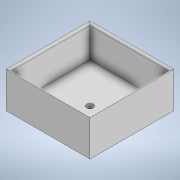
# Autodesk Inventor part: KwadratP
Saved by Autodesk Inventor 2020.3 (Build 243373000, 373)
## iProperties
Created: 2021-05-21
Part Number: KwadratP
Material: Generic
Document SubType Name: Modeling
Designer: patry
Density: 1 g/cm^3
Appearance: Default
Author: patry
Autodesk Inventor part; units mm, degrees
ref_plane "YZ Plane" through (0, 0, 0) normal (1, 0, 0) x (0, 1, 0)
ref_plane "XZ Plane" through (0, 0, 0) normal (0, 1, 0) x (-1, 0, 0)
ref_plane "XY Plane" through (0, 0, 0) normal (0, 0, 1) x (1, 0, 0)
sketch "Sketch1" plane through (0, 0, 0) normal (0, 1, 0) x (-1, 0, 0)
  line L0 (-52.5, -52.5) -> (52.5, -52.5)
  line L1 (52.5, -52.5) -> (52.5, 52.5)
  line L2 (52.5, 52.5) -> (-52.5, 52.5)
  line L3 (-52.5, 52.5) -> (-52.5, -52.5)
  line L4 (-52.5, -52.5) -> (52.5, 52.5) construction
  line L5 (52.5, -52.5) -> (-52.5, 52.5) construction
  point P0 (0, 0)
  constraints: 12 end point, 2 parallel, 1 horizontal, 1 perpendicular
extrude "Extrusion1" add sketch "Sketch1" along normal blind 5
sketch "Sketch4" plane through (0, 5, 0) normal (0, 1, 0) x (1, 0, 0)
  line L0 (-52.5, 52.5) -> (-52.5, -52.5) projected
  line L1 (52.5, 52.5) -> (-52.5, 52.5)
  line L2 (-52.5, 52.5) -> (-52.5, -52.5)
  line L3 (-52.5, -52.5) -> (52.5, -52.5)
  line L4 (52.5, -52.5) -> (52.5, 52.5)
  line L5 (52.5, 52.5) -> (-52.5, -52.5) construction
  line L6 (-52.5, 52.5) -> (52.5, -52.5) construction
  line L7 (50, 50) -> (-50, 50)
  line L8 (-50, 50) -> (-50, -50)
  line L9 (-50, -50) -> (50, -50)
  line L10 (50, -50) -> (50, 50)
  line L11 (50, 50) -> (-50, -50) construction
  line L12 (-50, 50) -> (50, -50) construction
  line L13 (52.5, 52.5) -> (-52.5, 52.5)
  line L14 (-52.5, 52.5) -> (-52.5, -52.5)
  line L15 (-52.5, -52.5) -> (52.5, -52.5)
  line L16 (52.5, -52.5) -> (52.5, 52.5)
  line L17 (52.5, 52.5) -> (-52.5, -52.5) construction
  line L18 (-52.5, 52.5) -> (52.5, -52.5) construction
  point P0 (0, 0)
  constraints: 36 end point, 6 midpoint, 6 parallel, 3 horizontal, 3 perpendicular
extrude "Extrusion2" add sketch "Sketch4" along normal blind 40
fillet "Fillet1" radius 2.5 4 edges at (0, 45, -50) (-50, 45, 0) (0, 45, 50) (50, 45, 0)
sketch "Sketch5" plane through (0, 5, 0) normal (0, 1, 0) x (1, 0, 0)
  circle A0 centre (0, 0) radius 2.5
  dimension "d12" = 5
  constraints: 1 centre point, 1 coincident
  measures "d12" diameter of A0
extrude "Extrusion3" cut sketch "Sketch5" against normal blind 10
sketch "Sketch6" plane through (0, 5, 0) normal (0, 1, 0) x (1, 0, 0)
  circle A0 centre (0, 0) radius 4.25
  dimension "d15" = 8.5
  constraints: 1 centre point, 1 coincident
  measures "d15" diameter of A0
extrude "Extrusion4" cut sketch "Sketch6" against normal blind 2
body "Solid1"
